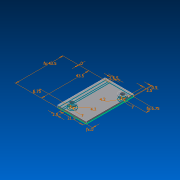
# Autodesk Inventor part: 12v regulator bracket
Saved by Autodesk Inventor 2015 (Build 190159000, 159)
## iProperties
Created: 2017-03-21
Part Number: 12v regulator bracket
Material: Generic
Document SubType Name: Modeling
Designer: ZigZagJoe
Density: 1 g/cm^3
Appearance: Default
Author: ZigZagJoe
Autodesk Inventor part; units mm, degrees
ref_plane "YZ Plane" through (0, 0, 0) normal (1, 0, 0) x (0, 1, 0)
ref_plane "XZ Plane" through (0, 0, 0) normal (0, 1, 0) x (-1, 0, 0)
ref_plane "XY Plane" through (0, 0, 0) normal (0, 0, 1) x (1, 0, 0)
sketch "Sketch1" plane through (0, 0, 0) normal (0, 0, 1) x (1, 0, 0)
  line L0 (-6.2577, 36.7396) -> (15.2423, 36.7396)
  line L1 (15.2423, 36.7396) -> (15.2423, -6.7604)
  line L2 (15.2423, -6.7604) -> (-6.2577, -6.7604)
  line L3 (-6.2577, -6.7604) -> (-6.2577, 36.7396)
  circle A0 centre (-3.7577, -0.0104) radius 2.1
  circle A1 centre (12.7423, 29.9896) radius 2.1
  circle A2 centre (12.7423, 29.9896) radius 3.5
  circle A3 centre (-3.7577, -0.0104) radius 3.5
  line L4 (-7.7577, 36.7396) -> (15.7423, 36.7396)
  line L5 (15.7423, 36.7396) -> (15.7423, -6.7604)
  line L6 (15.7423, -6.7604) -> (-7.7577, -6.7604)
  line L7 (-7.7577, -6.7604) -> (-7.7577, 36.7396)
  line L8 (-7.7577, -6.7604) -> (-10.2577, -6.7604)
  line L9 (-10.2577, -6.7604) -> (-10.2577, 36.7396)
  line L10 (-10.2577, 36.7396) -> (-7.7577, 36.7396)
  line L11 (-7.7577, 36.7396) -> (-7.7577, -6.7604)
  point P0 (0, 0)
  dimension "d0" = 21.5
  dimension "d1" = 43.5
  dimension "d2" = 6.75
  dimension "d3" = 6.75
  dimension "d4" = 2.5
  dimension "d5" = 2.5
  dimension "d6" = 7
  dimension "d7" = 7
  dimension "d8" = 0
  dimension "d9" = 1.5
  dimension "d10" = 0.5
  dimension "d11" = 0
  dimension "d12" = 2.5
  dimension "d20" = 4.2
  dimension "d21" = 4.2
  dimension "d22" = 43.5
  constraints: 24 end point, 6 parallel, 4 centre point, 3 horizontal, 3 perpendicular, 2 coincident
  measures "d0" distance of L1.end L2.end
  measures "d1" distance of L2.end L0.start
  measures "d2" distance from line of L0 A1.centre
  measures "d3" distance from line of L2 A0.centre
  measures "d4" distance from line of L3 A0.centre
  measures "d5" distance from line of L1 A1.centre
  measures "d6" diameter of A2
  measures "d7" diameter of A3
  measures "d8" distance between parallel lines of L4 L0
  measures "d9" distance between parallel lines of L3 L7
  measures "d10" distance between parallel lines of L5 L1
  measures "d11" distance between parallel lines of L2 L6
  measures "d12" distance of L9.end L10.end
  measures "d20" diameter of A0
  measures "d21" diameter of A1
  measures "d22" distance of L8.end L9.end
extrude "Extrusion1" add sketch "Sketch1" along normal blind 2
extrude "Extrusion2" [suppressed]
extrude "Extrusion3" add sketch "Sketch1" along normal blind 4 contours A3 L3 | L3 A3 | A2 L5 L1 | L1 A2 | A2 L5
fillet "Fillet1" [suppressed]
equation "\"d2\" = d3"
equation "\"d22\" = d1"
body "Solid1"
